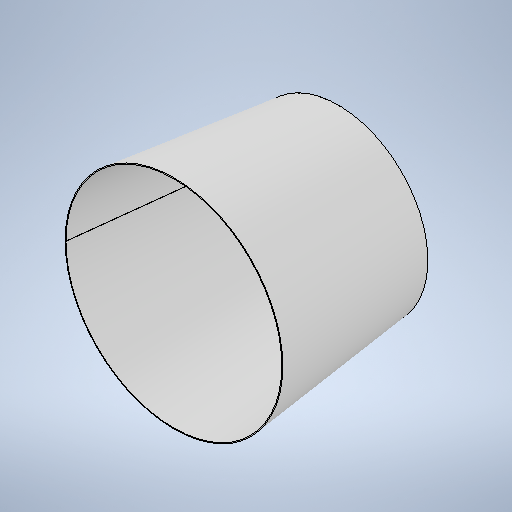
# Autodesk Inventor part: MSC 101 roсket tail
Saved by Autodesk Inventor 2025.1 (Build 291241020, 241B)
## iProperties
Created: 2024-05-19
Part Number: MSC 101 roсket tail
Material: Stainless Steel
Document SubType Name: Sheet Metal
Designer: admin
Density: 8 g/cm^3
Appearance: Default
Flat Pattern Width: 57.2191 cm
Flat Pattern Length: 33.0398 cm
Flat Pattern Area: 1890.51 cm^2
Sheet Metal Rule: Default
Sheet Metal Width: 572.191 mm
Sheet Metal Length: 330.398 mm
Sheet Metal Area: 189050.908 mm^2
Stock Number: МОО 101 ракета хвост
Mass: 478.711 g
Surface Area: 1507.2 cm^2
Volume: 59.8389 cm^3
Author: admin
Autodesk Inventor part; units mm, degrees
ref_plane "YZ Plane" through (0, 0, 0) normal (1, 0, 0) x (0, 1, 0)
ref_plane "XZ Plane" through (0, 0, 0) normal (0, 1, 0) x (-1, 0, 0)
ref_plane "XY Plane" through (0, 0, 0) normal (0, 0, 1) x (1, 0, 0)
sketch "Sketch1" plane through (0, 0, 0) normal (0, 0, 1) x (1, 0, 0)
  line L0 (0, 0) -> (0, 151)
  line L1 (-82.5, 151) -> (-100, 0.0922)
  line L2 (-100, 0.0922) -> (-99.2053, 0)
  line L3 (-99.2053, 0) -> (-81.7053, 150.9078)
  line L4 (-81.7053, 150.9078) -> (-82.5, 151)
  line L5 (-82.5, 151) -> (-99.2053, 0) construction
  line L6 (-100, 0.0922) -> (-81.7053, 150.9078) construction
  point P0 (-90.8527, 75.5)
  dimension "d0" = 151
  dimension "d4" = 200
  dimension "d6" = 165
  dimension "d7" = 0.8
  constraints: 14 end point, 2 horizontal alignment, 2 midpoint, 2 parallel, 1 perpendicular, 1 vertical
  measures "d0" distance of L0.start L0.end
  measures "d4" diameter of L1.end L0
  measures "d6" diameter of L1.start L0
  measures "d7" distance of L3.end L1.start
revolve "Revolution1" add sketch "Sketch1" angle 359.9 about axis through (0, 0, 0) along (0, 1, 0)
equation "\"d7\" = Thickness"
equation "\"BendRadius\" = Thickness"
equation "\"BendReliefWidth\" = Thickness"
equation "\"BendReliefDepth\" = 0.5 * Thickness"
equation "\"CornerReliefSize\" = 4 * Thickness"
equation "\"MinimumRemnant\" = 2 * Thickness"
equation "\"TransitionRadius\" = BendRadius"
equation "\"JacobiRadiusSize\" = BendRadius"
equation "\"GapSize\" = Thickness"
equation "\"Thickness\" = 0.8"
body "Solid1"
